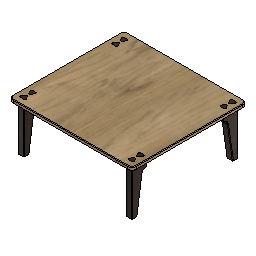
model (Autodesk Fusion 360 design; units mm, degrees)
Autodesk Fusion 360 part; units mm, degrees
sketch "tenon" plane through (0, 0, 0) normal (0, 0, 1) x (1, 0, 0)
  line L0 (15, 15) -> (65, 15)
  line L1 (65, 15) -> (65, 36.3)
  line L2 (65, 36.3) -> (15, 36.3)
  line L3 (15, 36.3) -> (15, 15)
  line L4 (19.699, 37.365) -> (19.699, 13.935) construction
  line L5 (19.699, 13.935) -> (39.99, 25.65) construction
  line L6 (39.99, 25.65) -> (19.699, 37.365) construction
  line L7 (19.699, 25.65) -> (15, 25.65) construction
  arc A0 (24.4615, 34.6154) -> (19.699, 31.8657) centre (22.874, 31.8657) ccw
  arc A1 (19.699, 19.4343) -> (24.4615, 16.6846) centre (22.874, 19.4343) ccw
  arc A2 (35.2275, 22.9004) -> (35.2275, 28.3996) centre (33.64, 25.65) ccw
  line L8 (19.699, 31.8657) -> (19.699, 19.4343)
  line L9 (24.4615, 16.6846) -> (35.2275, 22.9004)
  line L10 (35.2275, 28.3996) -> (24.4615, 34.6154)
  line L11 (40, 36.3) -> (40, 15) construction
  arc A3 (55.5385, 16.6846) -> (60.301, 19.4343) centre (57.126, 19.4343) ccw
  line L12 (55.5385, 16.6846) -> (44.7725, 22.9004)
  arc A4 (44.7725, 28.3996) -> (44.7725, 22.9004) centre (46.36, 25.65) ccw
  line L13 (44.7725, 28.3996) -> (55.5385, 34.6154)
  line L14 (60.301, 31.8657) -> (60.301, 19.4343)
  arc A5 (60.301, 31.8657) -> (55.5385, 34.6154) centre (57.126, 31.8657) ccw
  dimension "d1" = 21.3
  dimension "d2" = 3.175
  dimension "d4" = 23.43
  dimension "d5" = 50
  dimension "d6" = 0.01
  dimension "d27" = 15
  dimension "d28" = 15
  constraint horizontal L2
  constraint equal L4 L5
  constraint equal L4 L6
  constraint midpoint L4 L7.start
  constraint midpoint L3 L7.end
  constraint tangent L6 A0
  constraint coincident L6 A0.start
  constraint coincident L4 A0.end
  constraint tangent L4 A0
  constraint tangent L4 A1
  constraint coincident L5 A1.end
  constraint coincident L4 A1.start
  constraint tangent L5 A2
  constraint coincident L6 A2.end
  constraint coincident L5 A2.start
  constraint tangent L6 A2
  constraint tangent L5 A1
  constraint equal A1 A2
  constraint equal A0 A2
  constraint tangent A2 L9
  constraint tangent A0 L10
  constraint midpoint L2 L11.start
  constraint midpoint L0 L11.end
  constraint symmetric A0.end L11 L14.start
  constraint symmetric A0.start L11 L13.end
  constraint symmetric A0 L11 A5
  constraint symmetric A1.start L11 A3.end
  constraint symmetric A1.end L11 A3.start
  constraint symmetric A1 L11 A3
  constraint symmetric A2.start L11 L12.end
  constraint symmetric A2.end L11 A4.start
  constraint symmetric A2 L11 A4
  constraint perpendicular L3 L7
  constraint perpendicular L0 L3
  constraint perpendicular L7 L8
  constraint perpendicular L1 L2
  constraint perpendicular L0 L1
  measures "d1" distance of L0.start L2.end
  measures "d2" radius of A0
  measures "d4" distance of L4.start L4.end
  measures "d5" distance of L1.end L2.end
  measures "d6" distance of L5.end L11
  measures "d27" vertical distance of origin L0.start
  measures "d28" horizontal distance of origin L0.start
sketch "top" plane through (0, 0, 0) normal (0, 0, 1) x (1, 0, 0)
  line L0 (0, 0) -> (416, 0)
  line L1 (416, 0) -> (416, 389)
  line L2 (416, 389) -> (0, 389)
  line L3 (0, 389) -> (0, 0)
  line L4 (0, 194.5) -> (416, 194.5) construction
  line L5 (208, 389) -> (208, 0) construction
  line L6 (15, 374) -> (36.3, 374)
  line L7 (36.3, 374) -> (36.3, 324)
  line L8 (36.3, 324) -> (15, 324)
  line L9 (15, 324) -> (15, 374)
  line L10 (401, 324) -> (401, 374)
  line L11 (401, 374) -> (379.7, 374)
  line L12 (379.7, 324) -> (401, 324)
  line L13 (379.7, 374) -> (379.7, 324)
  line L14 (15, 65) -> (15, 15)
  line L15 (15, 15) -> (36.3, 15)
  line L16 (36.3, 65) -> (15, 65)
  line L17 (36.3, 15) -> (36.3, 65)
  line L18 (401, 65) -> (401, 15)
  line L19 (401, 15) -> (379.7, 15)
  line L20 (379.7, 65) -> (401, 65)
  line L21 (379.7, 15) -> (379.7, 65)
  dimension "d7" = 389
  dimension "d8" = 416
  dimension "d9" = 21.3
  dimension "d10" = 50
  dimension "d11" = 15
  dimension "d12" = 15
  constraint horizontal L0
  constraint vertical L1
  constraint horizontal L2
  constraint vertical L3
  constraint coincident L0.start L3.end
  constraint midpoint L3 L4.start
  constraint midpoint L1 L4.end
  constraint midpoint L2 L5.start
  constraint midpoint L0 L5.end
  constraint horizontal L6
  constraint vertical L7
  constraint horizontal L8
  constraint vertical L9
  constraint symmetric L5 L6.start L10.end
  constraint symmetric L5 L6.end L11.end
  constraint symmetric L5 L7.end L12.start
  constraint symmetric L5 L8.end L10.start
  constraint symmetric L4 L6.start L14.end
  constraint symmetric L4 L6.end L15.end
  constraint symmetric L4 L7.end L16.start
  constraint symmetric L4 L8.end L14.start
  constraint symmetric L4 L10.start L18.start
  constraint symmetric L4 L10.end L18.end
  constraint symmetric L4 L11.end L19.end
  constraint symmetric L4 L12.start L20.start
  measures "d7" distance of L0.start L2.end
  measures "d8" distance of L1.end L2.end
  measures "d9" distance of L6.start L6.end
  measures "d10" distance of L6.start L8.end
  measures "d11" vertical distance of L2.end L6.start
  measures "d12" horizontal distance of L2.end L6.start
extrude "Extrude1" add sketch "top" along normal blind 18 contours L0 L1 L2 L3 | L6 L7 L8 L9 | L10 L11 L12 L13 | L14 L15 L16 L17 | L18 L19 L20 L21 makes body 1
extrude "Extrude2" add sketch "top" against normal blind 149 separate body contours L14 L15 L16 L17 makes body 2
extrude "Extrude4" add sketch "tenon" along normal up to surface (18 mm away) separate body contours A0 A1 A2 L8 L9 L10 | A3 L12 A4 L13 L14 A5 makes body 3 at (19.699, 27.7219, 6) makes body 4 at (60.301, 27.7219, 6)
move_body "Move1" bodies 3 4 to x (0, 1, 0) y (-1, 0, 0) z (0, 0, 1) at (51.207, -0.607, 0)
combine "Combine1" operation add target body 2 tool bodies 4 3
fillet "Fillet1" radius 15 4 edges at (0, 0, 9) (416, 0, 9) (416, 389, 9) (0, 389, 9) on bodies 1
sketch "leg" plane through (15, 0, 0) normal (-1, 0, 0) x (0, -1, 0)
  line L0 (-15, 0) -> (-65, 0)
  line L1 (-65, 0) -> (-65, -149)
  line L2 (-65, -149) -> (-15, -149)
  line L3 (-15, -149) -> (-15, 0)
  line L4 (-33, -149) -> (-50.1658, -30.8434)
  arc A0 (-50.1658, -30.8434) -> (-65, -18) centre (-65.01, -33) ccw
  line L5 (-374, 0) -> (-15, 0)
  dimension "d19" = 18
  dimension "d20" = 18
  dimension "d21" = 15
  dimension "d22" = 0.01
  constraint coincident L2 L4.start
  constraint coincident L1 A0.end
  constraint tangent L4 A0
  measures "d19" distance of L2.end L4.start
  measures "d20" distance of L0.end A0.end
  measures "d21" radius of A0
  measures "d22" horizontal distance of A0.end A0.centre
extrude "Extrude3" cut sketch "leg" against normal up to surface (21.3 mm away) contours L1 L2 L4 A0 bodies 2
chamfer "Chamfer1" distance 8 angle 45 8 edges at (208, 0, 0) (411.6066, 4.3934, 0) (416, 194.5, 0) (411.6066, 384.6066, 0) (208, 389, 0) (4.3934, 384.6066, 0) (0, 194.5, 0) (4.3934, 4.3934, 0) on bodies 1 2
chamfer "Chamfer1" distance 2 angle 45 14 edges at (15, 15, -74.5) (36.3, 15, -74.5) (15, 41.5829, -89.9217) (15, 55.1917, -21.6598) (36.3, 41.5829, -89.9217) (36.3, 55.1917, -21.6598) (208, 389, 18) (4.3934, 384.6066, 18) (0, 194.5, 18) (4.3934, 4.3934, 18) (208, 0, 18) (411.6066, 4.3934, 18) (416, 194.5, 18) (411.6066, 384.6066, 18) 1 faces at (22.1, 27, -149) on bodies 1 2
ref_plane "WorkPlane1" through (208, 194.5, 12) normal (-1, 0, 0) x (0, -1, 0)
ref_plane "WorkPlane2" through (208, 194.5, 12) normal (0, -1, 0) x (1, 0, 0)
mirror "Mirror1" about plane through (208, 194.5, 12) normal (-1, 0, 0) of bodies 2 makes body 5
mirror "Mirror2" about plane through (208, 194.5, 12) normal (0, -1, 0) of bodies 2 5 makes body 6 at (15, 361.6045, -59.1853) makes body 7 at (401, 361.6045, -59.1853)
combine "Combine2" operation cut target body 1 tool bodies 2 5 7 6 keep tools
equation "d2 = 1/4\" / 2"
equation "d4 = d1 * 1.1"
equation "d12 = d11"
equation "d15 = -167 mm + 18 mm"
named bodies: "top", "leg1", "leg2", "leg3", "leg4"
